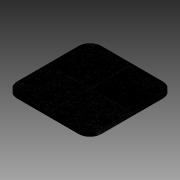
# Autodesk Inventor part: basalt
Saved by Autodesk Inventor 2014 (Build 180170000, 170)
## iProperties
Created: 2013-07-23
Part Number: basalt
Material: Generic
Document SubType Name: Modeling
Designer: employee
Density: 1 g/cm^3
Mass: 472.881 g
Surface Area: 1083.44 cm^2
Volume: 472.881 cm^3
Appearance: Polished - Black
Author: employee
Autodesk Inventor part; units mm, degrees
ref_plane "YZ Plane" through (0, 0, 0) normal (1, 0, 0) x (0, 1, 0)
ref_plane "XZ Plane" through (0, 0, 0) normal (0, 1, 0) x (-1, 0, 0)
ref_plane "XY Plane" through (0, 0, 0) normal (0, 0, 1) x (1, 0, 0)
sketch "Sketch1" plane through (0, 0, 0) normal (0, 0, 1) x (1, 0, 0)
  circle A0 centre (0, 0) radius 100 construction
  line L0 (112.5, 0) -> (112.5, 112.5)
  line L1 (112.5, 112.5) -> (-112.5, 112.5)
  line L2 (-112.5, 112.5) -> (-112.5, -112.5)
  line L3 (-112.5, -112.5) -> (112.5, -112.5)
  line L4 (112.5, -112.5) -> (112.5, 0)
  circle A1 centre (-75, -100) radius 4.05
  circle A2 centre (75, -100) radius 4.05
  line L5 (75, -100) -> (-75, -100) construction
  line L6 (-75, -100) -> (-75, 100) construction
  line L7 (-75, 100) -> (75, 100) construction
  line L8 (75, 100) -> (75, -100) construction
  circle A3 centre (-75, 100) radius 4.05
  circle A4 centre (75, 100) radius 4.05
  point P0 (0, 112.5)
  point P1 (75, 0)
  dimension "d0" = 200
  dimension "d2" = 225
  dimension "d3" = 225
  dimension "d4" = 150
  dimension "d5" = 37.5
  dimension "d6" = 12.5
  dimension "d7" = 8.1
  constraints: 18 end point, 5 centre point, 4 coincident, 4 parallel, 3 equal radius, 3 horizontal alignment, 2 collinear, 2 midpoint, 2 perpendicular, 1 horizontal, 1 vertical, 1 vertical alignment
  measures "d0" diameter of A0
  measures "d2" distance of L0.end L1.end
  measures "d3" distance between parallel lines of L3 L1
  measures "d4" distance of L5.start A1.centre
  measures "d5" distance from line of A1.centre L2
  measures "d6" distance from line of A1.centre L3
  measures "d7" diameter of A1
extrude "Extrusion1" add sketch "Sketch1" along normal blind 9.525
fillet "Fillet1" radius 30 4 edges at (-112.5, -112.5, 4.7625) (-112.5, 112.5, 4.7625) (112.5, -112.5, 4.7625) (112.5, 112.5, 4.7625)
body "Solid1"
